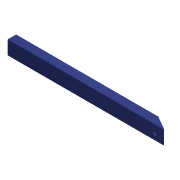
# Autodesk Inventor part: Barra nuevo pivote
Saved by Autodesk Inventor 2019 (Build 230136000, 136)
## iProperties
Created: 2020-02-07
Part Number: Barra nuevo pivote
Material: Generic
Document SubType Name: Modeling
Designer: Juan Carlos Botero
Density: 1 g/cm^3
Appearance: 48,59,150
Author: Juan Carlos Botero
Autodesk Inventor part; units mm, degrees
ref_plane "YZ Plane" through (0, 0, 0) normal (1, 0, 0) x (0, 1, 0)
ref_plane "XZ Plane" through (0, 0, 0) normal (0, 1, 0) x (-1, 0, 0)
ref_plane "XY Plane" through (0, 0, 0) normal (0, 0, 1) x (1, 0, 0)
sketch "Sketch1" plane through (0, 0, 0) normal (0, 0, 1) x (1, 0, 0)
  line L0 (-651.5983, 84.4921) -> (440.9045, 84.4921)
  line L1 (440.9045, 84.4921) -> (440.9045, -15.5079)
  line L2 (440.9045, -15.5079) -> (-651.5983, -15.5079)
  line L3 (-651.5983, -15.5079) -> (-651.5983, 84.4921)
  line L4 (-651.5983, -15.5079) -> (-899.2765, -81.873) projected
  point P0 (0, 0)
  dimension "d0" = 100
  constraints: 8 end point, 2 parallel, 1 horizontal, 1 perpendicular, 1 point on line
  measures "d0" distance of L0.end L1.end
extrude "Extrusion1" add sketch "Sketch1" against normal blind 60
fillet "Fillet1" radius 3 4 edges at (-105.3469, 84.4921, 0) (-105.3469, 84.4921, -60) (-105.3469, -15.5079, 0) (-105.3469, -15.5079, -60)
shell "Shell1" thickness 3 removed faces 2 at (440.9045, 18.8255, -40) at (-651.5983, 18.8255, -40)
sketch "Sketch2" plane through (0, 0, 0) normal (0, 0, 1) x (1, 0, 0)
  circle A0 centre (377.8245, 22.8431) radius 11.25 projected
  point P0 (0, 0)
extrude "Extrusion2" cut sketch "Sketch2" against normal through all
sketch "Sketch3" plane through (-651.5983, 84.4921, -57) normal (0, 1, 0) x (1, 0, 0)
  line L0 (0, 0) -> (1092.5029, 0) projected
  line L1 (0, -54) -> (0, 0) projected
  line L2 (1092.5029, -54) -> (0, -54) projected
  line L3 (1092.5029, -54) -> (1092.5029, 0) projected
  line L4 (1092.5029, -54) -> (998.9721, 0)
  line L5 (0, 0) -> (1092.5029, 0) projected
  line L6 (1092.5029, -54) -> (1101.6667, -54)
  line L7 (1101.6667, -54) -> (1101.6667, 18.4263)
  line L8 (1101.6667, 18.4263) -> (998.9721, 18.4263)
  line L9 (998.9721, 18.4263) -> (998.9721, 0)
  point P0 (651.5983, -57)
  dimension "d8" = 30
  constraints: 10 end point, 3 perpendicular, 1 horizontal, 1 point on line
  measures "d8" angle of L2 L4
extrude "Extrusion3" cut sketch "Sketch3" against normal through all contours L9 L8 L7 L6 L3 L0 | L0 L3 L4
body "Solid1"
